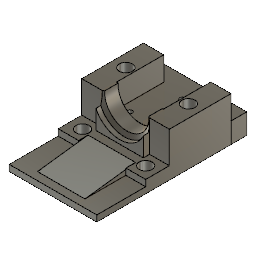
camera-mount v2 (Autodesk Fusion 360 design; units mm, degrees)
Autodesk Fusion 360 part; units mm, degrees
sketch "Sketch1" plane through (0, 0, 0) normal (0, 0, 1) x (1, 0, 0)
  line L0 (0, 0) -> (30, 0)
  line L1 (30, 0) -> (30, 30)
  line L2 (30, 30) -> (0, 30)
  line L3 (0, 30) -> (0, 0)
  circle A0 centre (15, 26.5) radius 1.5
  circle A1 centre (5.5, 3) radius 1.5
  circle A2 centre (24.5, 3) radius 1.5
  dimension "d2" = 3
  dimension "d3" = 5.5
  dimension "d5" = 5.5
  dimension "d6" = 3
  dimension "d8" = 15
  dimension "d9" = 3.5
  dimension "d17" = 3
  dimension "d18" = 3
  dimension "d19" = 3
  constraint horizontal L0
  constraint vertical L1
  constraint horizontal L2
  constraint vertical L3
  constraint coincident L0.start L3.end
  measures "d2" distance of L0 A1.centre
  measures "d3" distance of L3 A1.centre
  measures "d5" distance of L1 A2.centre
  measures "d6" distance of L0 A2.centre
  measures "d8" distance of L3 A0.centre
  measures "d9" distance of L2 A0.centre
  measures "d17" diameter of A0
  measures "d18" diameter of A1
  measures "d19" diameter of A2
extrude "Extrude1" add sketch "Sketch1" along normal blind 13
sketch "Sketch2" plane through (0, 0, 0) normal (0, 0, 1) x (1, 0, 0)
sketch "Sketch3" plane through (0, 0, 0) normal (0, 0, 1) x (1, 0, 0)
chamfer "Chamfer1" distance 1.5 angle 45 1 edges at (4.1015, 3.5424, 0)
chamfer "Chamfer2" distance 1.5 angle 45 1 edges at (13.6015, 27.0424, 0)
chamfer "Chamfer3" distance 1.5 angle 45 1 edges at (23.1015, 3.5424, 0)
sketch "Sketch4" plane through (0, 0, 0) normal (0, 0, 1) x (1, 0, 0)
  line L0 (0, 0) -> (30, 0)
  line L1 (30, 0) -> (30, -10)
  line L2 (30, -10) -> (0, -10)
  line L3 (0, -10) -> (0, 0)
  dimension "d25" = 10
  dimension "d26" = 30
  constraint horizontal L0
  constraint vertical L1
  constraint horizontal L2
  constraint vertical L3
  constraint coincident L0.start L3.end
  measures "d25" distance of L0.start L2.end
  measures "d26" distance of L1.end L2.end
extrude "Extrude2" add sketch "Sketch4" along normal blind 28
sketch "Sketch5" plane through (0, -10, 0) normal (0, -1, 0) x (1, 0, 0)
  line L0 (0, 0) -> (30, 0)
  line L1 (30, 0) -> (30, 28)
  line L2 (30, 28) -> (0, 28)
  line L3 (0, 28) -> (0, 0)
  circle A0 centre (15, 27) radius 14
  dimension "d29" = 28
  dimension "d30" = 27
  measures "d29" diameter of A0
  measures "d30" distance of L0 A0.centre
extrude "Extrude3" cut sketch "Sketch5" against normal blind 10 contours L2 A0 picked at (14.1563, 23.0769)
sketch "Sketch6" plane through (0, 0, 0) normal (-1, 0, 0) x (0, -1, 0)
  line L0 (-30, 0) -> (10, 0)
  line L1 (10, 0) -> (10, 28)
  line L2 (10, 28) -> (0, 28)
  line L3 (0, 28) -> (0, 13)
  line L4 (0, 13) -> (-30, 13)
  line L5 (-30, 13) -> (-30, 0)
sketch "Sketch7" plane through (0, 0, 0) normal (0, 0, 1) x (1, 0, 0)
  line L0 (0, -10) -> (30, -10)
  line L1 (30, -10) -> (30, -55)
  line L2 (30, -55) -> (0, -55)
  line L3 (0, -55) -> (0, -10)
  dimension "d33" = 30
  dimension "d34" = 45
  constraint horizontal L0
  constraint vertical L1
  constraint horizontal L2
  constraint vertical L3
  measures "d33" distance of L0.start L0.end
  measures "d34" distance of L0.start L2.end
extrude "Extrude4" add sketch "Sketch7" along normal blind 4
sketch "Sketch8" plane through (0, 0, 0) normal (0, 0, 1) x (1, 0, 0)
  line L0 (0, -10) -> (30, -10)
  line L1 (30, -10) -> (30, -13)
  line L2 (30, -13) -> (0, -13)
  line L3 (0, -13) -> (0, -10)
  dimension "d37" = 3
  constraint horizontal L0
  constraint vertical L1
  constraint horizontal L2
  constraint vertical L3
  measures "d37" distance of L0.start L2.end
extrude "Extrude5" add sketch "Sketch8" along normal blind 28
sketch "Sketch9" plane through (30, 0, 0) normal (1, 0, 0) x (0, 1, 0)
  line L0 (-13, 4) -> (-55, 4)
  line L1 (-55, 4) -> (-55, 0)
  line L2 (-55, 0) -> (30, 0)
  line L3 (30, 0) -> (30, 13)
  line L4 (30, 13) -> (0, 13)
  line L5 (0, 13) -> (0, 28)
  line L6 (0, 28) -> (-13, 28)
  line L7 (-13, 28) -> (-13, 4)
hole "Hole1" at (15, -13, 27) direction (0, 1, 0) diameter 33 depth 3 tip angle 118
sketch "Sketch10" plane through (0, 0, 4) normal (0, 0, 1) x (-1, 0, 0)
  line L0 (-30, 13) -> (0, 13)
  line L1 (0, 13) -> (0, 55)
  line L2 (0, 55) -> (-30, 55)
  line L3 (-30, 55) -> (-30, 13)
  line L4 (0, 55) -> (-30, 55)
  line L5 (-30, 55) -> (-30, 50)
  line L6 (-30, 50) -> (0, 50)
  line L7 (0, 50) -> (0, 55)
  dimension "d45" = 5
  constraint horizontal L4
  constraint vertical L5
  constraint horizontal L6
  constraint vertical L7
  constraint coincident L3 L5.end
  constraint coincident L1.end L2.start
  measures "d45" distance of L1.end L6.end
extrude "Extrude6" cut sketch "Sketch10" against normal blind 4 contours L1 L2 L3 L4 L5 L6 L7
sketch "Sketch11" plane through (0, 0, 4) normal (0, 0, 1) x (-1, 0, 0)
  line L0 (0, 50) -> (-30, 50)
  line L1 (-30, 50) -> (-30, 13)
  line L2 (-30, 13) -> (0, 13)
  line L3 (0, 13) -> (0, 50)
  line L4 (0, 13) -> (-30, 13)
  line L5 (-30, 13) -> (-30, 18)
  line L6 (-30, 18) -> (0, 18)
  line L7 (0, 18) -> (0, 13)
  dimension "d48" = 30
  dimension "d49" = 5
  constraint horizontal L4
  constraint vertical L5
  constraint horizontal L6
  constraint vertical L7
  constraint coincident L2.end L3.start
  measures "d48" distance of L2.end L1.end
  measures "d49" distance of L2.end L6.end
extrude "Extrude7" add sketch "Sketch11" along normal blind 4 contours L1 L2 L3 L4 L5 L6 L7
loft "Loft1" add section 1 face at (20, -18, 5.3333) section 2 face at (20, -50, 2.6667)
sketch "Sketch12" plane through (0, 0, 0) normal (0, 0, 1) x (1, 0, 0)
  line L0 (0, -50) -> (30, -50)
  line L1 (30, -50) -> (30, -55)
  line L2 (30, -55) -> (0, -55)
  line L3 (0, -55) -> (0, -50)
  constraint horizontal L0
  constraint vertical L1
  constraint horizontal L2
  constraint vertical L3
extrude "Extrude8" add sketch "Sketch12" along normal blind 4
sketch "Sketch13" plane through (0, 0, 0) normal (0, 0, 1) x (1, 0, 0)
  line L0 (0, 30) -> (-13, 30)
  line L1 (-13, 30) -> (-13, -9.1)
  line L2 (-13, -9.1) -> (0, -9.1)
  line L3 (0, -9.1) -> (0, 30)
  line L4 (29.6458, 30) -> (42.6458, 30)
  line L5 (42.6458, 30) -> (42.6458, -9.1)
  line L6 (42.6458, -9.1) -> (29.6458, -9.1)
  line L7 (29.6458, -9.1) -> (29.6458, 30)
  circle A0 centre (-5, 10.9) radius 4.1
  circle A1 centre (34.6458, 10.9) radius 4.1
  dimension "d54" = 13
  dimension "d55" = 8.2
  dimension "d56" = 8.2
  dimension "d58" = 5
  dimension "d59" = 13
  dimension "d60" = 5
  dimension "d61" = 20
  dimension "d62" = 39.1
  dimension "d63" = 39.1
  dimension "d64" = 20
  constraint horizontal L0
  constraint vertical L1
  constraint horizontal L2
  constraint vertical L3
  constraint horizontal L4
  constraint vertical L5
  constraint horizontal L6
  constraint vertical L7
  measures "d54" distance of L0.start L0.end
  measures "d55" diameter of A0
  measures "d56" diameter of A1
  measures "d58" distance of L3 A0.centre
  measures "d59" distance of L4.start L4.end
  measures "d60" distance of L7 A1.centre
  measures "d61" distance of L6 A1.centre
  measures "d62" distance of L4.end L5.end
  measures "d63" distance of L0.end L1.end
  measures "d64" distance of L2 A0.centre
extrude "Extrude9" add sketch "Sketch13" along normal blind 28
sketch "Sketch14" plane through (0, 0, 0) normal (1, 0, 0) x (0, 1, 0)
sketch "Sketch15" plane through (0, 0, 0) normal (0, 0, 1) x (1, 0, 0)
  line L0 (0, -9) -> (-13, -9)
  line L1 (-13, -9) -> (-13, -24)
  line L2 (-13, -24) -> (0, -24)
  line L3 (0, -24) -> (0, -9)
  circle A0 centre (-5, -16.5) radius 4.1
  line L4 (42.645, -9.1) -> (30, -9.1)
  line L5 (30, -9.1) -> (30, -24.1)
  line L6 (30, -24.1) -> (42.645, -24.1)
  line L7 (42.645, -24.1) -> (42.645, -9.1)
  circle A1 centre (35, -16.6) radius 4.1
  dimension "d67" = 13
  dimension "d68" = 8.2
  dimension "d69" = 15
  dimension "d70" = 12.645
  dimension "d71" = 8.2
  dimension "d72" = 5
  dimension "d73" = 7.5
  dimension "d74" = 15
  dimension "d75" = 7.5
  dimension "d76" = 5
  constraint horizontal L0
  constraint vertical L1
  constraint horizontal L2
  constraint vertical L3
  constraint horizontal L4
  constraint vertical L5
  constraint horizontal L6
  constraint vertical L7
  measures "d67" distance of L1.end L2.end
  measures "d68" diameter of A0
  measures "d69" distance of L4.start L6.end
  measures "d70" distance of L5.end L6.end
  measures "d71" diameter of A1
  measures "d72" distance of L3 A0.centre
  measures "d73" distance of L0 A0.centre
  measures "d74" distance of L0.end L1.end
  measures "d75" distance of L4 A1.centre
  measures "d76" distance of L5 A1.centre
extrude "Extrude10" add sketch "Sketch15" along normal blind 8
sketch "Sketch16" plane through (0, 0, 0) normal (0, 0, 1) x (1, 0, 0)
  line L0 (-13, -24) -> (0, -24)
  line L1 (0, -24) -> (0, -55)
  line L2 (0, -55) -> (-13, -55)
  line L3 (-13, -55) -> (-13, -24)
  line L4 (42.6, -24.1) -> (30, -24.1)
  line L5 (30, -24.1) -> (30, -55.1)
  line L6 (30, -55.1) -> (42.6, -55.1)
  line L7 (42.6, -55.1) -> (42.6, -24.1)
  dimension "d79" = 31
  constraint horizontal L0
  constraint vertical L1
  constraint horizontal L2
  constraint vertical L3
  constraint horizontal L4
  constraint vertical L5
  constraint horizontal L6
  constraint vertical L7
  measures "d79" distance of L4.start L6.end
extrude "Extrude11" add sketch "Sketch16" along normal blind 4
sketch "Sketch17" plane through (0, 0, 0) normal (0, 0, 1) x (1, 0, 0)
  line L0 (-13, -55) -> (43, -55)
  line L1 (43, -55) -> (43, -56)
  line L2 (43, -56) -> (-13, -56)
  line L3 (-13, -56) -> (-13, -55)
  constraint horizontal L0
  constraint vertical L1
  constraint horizontal L2
  constraint vertical L3
extrude "Extrude12" cut sketch "Sketch17" along normal blind 5
sketch "Sketch18" plane through (0, 0, 0) normal (0, 0, 1) x (1, 0, 0)
  line L0 (42.5262, -55.0015) -> (61.8267, -55.0015)
  line L1 (61.8267, -55.0015) -> (61.8267, 35.7462)
  line L2 (61.8267, 35.7462) -> (42.5262, 35.7462)
  line L3 (42.5262, 35.7462) -> (42.5262, -55.0015)
  constraint horizontal L0
  constraint vertical L1
  constraint horizontal L2
  constraint vertical L3
extrude "Extrude13" cut sketch "Sketch18" along normal blind 30
sketch "Sketch19" plane through (0, 0, 0) normal (0, 0, 1) x (1, 0, 0)
  line L0 (-13, 30) -> (42.5, 30)
  line L1 (42.5, 30) -> (42.5, 40)
  line L2 (42.5, 40) -> (-13, 40)
  line L3 (-13, 40) -> (-13, 30)
  dimension "d86" = 10
  constraint horizontal L0
  constraint vertical L1
  constraint horizontal L2
  constraint vertical L3
  measures "d86" distance of L0.end L1.end
extrude "Extrude14" add sketch "Sketch19" along normal blind 13
